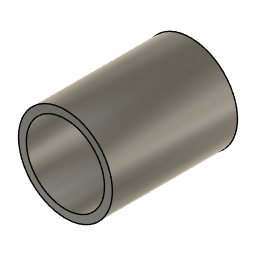
TANK v2 (Autodesk Fusion 360 archive; units mm, degrees)
design "Nozzle"
Autodesk Fusion 360 part; units mm, degrees
sketch "Sketch1" plane through (0, 0, 0) normal (0, 1, 0) x (1, 0, 0)
  circle A0 centre (0, 0) radius 12.5
  circle A1 centre (0, 0) radius 15
  dimension "d1" = 25
  dimension "d2" = 30
  constraint coincident A0.centre A1.centre
  constraint concentric A0 A1
  measures "d1" diameter of A0
  measures "d2" diameter of A1
extrude "Extrude1" add sketch "Sketch1" along normal blind 40

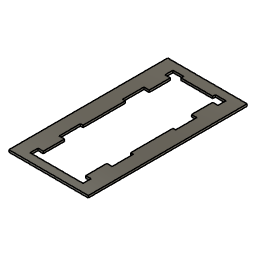
design "Potoboard holder"
Autodesk Fusion 360 part; units mm, degrees
sketch "Sketch1" plane through (0, 0, 0) normal (0, 0, 1) x (1, 0, 0)
  line L0 (-75, 150) -> (75, 150)
  line L1 (75, 150) -> (75, -150)
  line L2 (75, -150) -> (-75, -150)
  line L3 (-75, -150) -> (-75, 150)
  line L4 (-75, 150) -> (75, -150) construction
  line L5 (75, 150) -> (-75, -150) construction
  line L6 (50, 135) -> (-50, 135)
  line L7 (-50, 135) -> (-50, -135)
  line L8 (-50, -135) -> (50, -135)
  line L9 (50, -135) -> (50, 135)
  line L10 (50, 135) -> (-50, -135) construction
  line L11 (-50, 135) -> (50, -135) construction
  line L12 (-30, 135) -> (30, 135)
  line L13 (30, 135) -> (30, 130)
  line L14 (30, 130) -> (-30, 130)
  line L15 (-30, 130) -> (-30, 135)
  line L16 (-50, 40) -> (-45, 40)
  line L17 (-45, 40) -> (-45, -40)
  line L18 (-45, -40) -> (-50, -40)
  line L19 (-50, -40) -> (-50, 40)
  line L20 (-30, -135) -> (30, -135)
  line L21 (30, -135) -> (30, -130)
  line L22 (30, -130) -> (-30, -130)
  line L23 (-30, -130) -> (-30, -135)
  line L24 (50, 40) -> (45, 40)
  line L25 (45, 40) -> (45, -40)
  line L26 (45, -40) -> (50, -40)
  line L27 (50, -40) -> (50, 40)
  line L28 (-50, -80) -> (-40, -80)
  line L29 (-40, -80) -> (-40, -120)
  line L30 (-40, -120) -> (-50, -120)
  line L31 (-50, -120) -> (-50, -80)
  line L32 (50, -120) -> (40, -120)
  line L33 (40, -120) -> (40, -80)
  line L34 (40, -80) -> (50, -80)
  line L35 (50, -80) -> (50, -120)
  line L36 (50, 120) -> (40, 120)
  line L37 (40, 120) -> (40, 80)
  line L38 (40, 80) -> (50, 80)
  line L39 (50, 80) -> (50, 120)
  line L40 (-50, 120) -> (-40, 120)
  line L41 (-40, 120) -> (-40, 80)
  line L42 (-40, 80) -> (-50, 80)
  line L43 (-50, 80) -> (-50, 120)
  dimension "d1" = 300
  dimension "d2" = 150
  dimension "d3" = 270
  dimension "d4" = 100
  dimension "d5" = 60
  dimension "d6" = 20
  dimension "d7" = 5
  dimension "d8" = 80
  dimension "d9" = 95
  dimension "d10" = 5
  dimension "d11" = 60
  dimension "d12" = 5
  dimension "d13" = 20
  dimension "d14" = 80
  dimension "d15" = 5
  dimension "d16" = 95
  dimension "d19" = 10
  dimension "d20" = 40
  dimension "d21" = 40
  dimension "d22" = 10
  dimension "d23" = 40
  dimension "d24" = 40
  dimension "d25" = 10
  dimension "d26" = 40
  dimension "d27" = 40
  dimension "d28" = 10
  dimension "d29" = 40
  dimension "d30" = 40
  constraint horizontal L0
  constraint perpendicular L0 L1
  constraint parallel L0 L2
  constraint parallel L1 L3
  constraint coincident L4 origin
  constraint coincident L5 origin
  constraint horizontal L6
  constraint perpendicular L6 L7
  constraint parallel L6 L8
  constraint parallel L7 L9
  constraint coincident L10 origin
  constraint coincident L11 origin
  constraint horizontal L12
  constraint vertical L13
  constraint horizontal L14
  constraint vertical L15
  constraint coincident L6 L12.start
  constraint horizontal L16
  constraint vertical L17
  constraint horizontal L18
  constraint vertical L19
  constraint coincident L7 L16.start
  constraint horizontal L20
  constraint vertical L21
  constraint horizontal L22
  constraint vertical L23
  constraint coincident L8 L20.start
  constraint horizontal L24
  constraint vertical L25
  constraint horizontal L26
  constraint vertical L27
  constraint coincident L9 L24.start
  constraint horizontal L28
  constraint vertical L29
  constraint horizontal L30
  constraint vertical L31
  constraint coincident L7 L28.start
  constraint horizontal L32
  constraint vertical L33
  constraint horizontal L34
  constraint vertical L35
  constraint coincident L9 L32.start
  constraint horizontal L36
  constraint vertical L37
  constraint horizontal L38
  constraint vertical L39
  constraint coincident L9 L36.start
  constraint horizontal L40
  constraint vertical L41
  constraint horizontal L42
  constraint vertical L43
  constraint coincident L7 L40.start
  measures "d1" distance of L0.start L2.end
  measures "d2" distance of L0.start L0.end
  measures "d3" distance of L6.end L7.end
  measures "d4" distance of L6.start L6.end
  measures "d5" distance of L13.end L14.end
  measures "d6" distance of L6.end L12.start
  measures "d7" distance of L12.end L13.end
  measures "d8" distance of L16.end L17.end
  measures "d9" distance of L6.end L16.start
  measures "d10" distance of L17.end L18.end
  measures "d11" distance of L21.end L22.end
  measures "d12" distance of L20.start L22.end
  measures "d13" distance of L7.end L20.start
  measures "d14" distance of L24.end L25.end
  measures "d15" distance of L24.start L24.end
  measures "d16" distance of L6.start L24.start
  measures "d19" distance of L28.start L28.end
  measures "d20" distance of L28.end L29.end
  measures "d21" distance of L18.end L28.start
  measures "d22" distance of L32.start L32.end
  measures "d23" distance of L32.end L33.end
  measures "d24" distance of L26.end L34.end
  measures "d25" distance of L36.start L36.end
  measures "d26" distance of L36.end L37.end
  measures "d27" distance of L24 L38.end
  measures "d28" distance of L40.start L40.end
  measures "d29" distance of L40.end L41.end
  measures "d30" distance of L16.start L42.end
extrude "Extrude2" add sketch "Sketch1" along normal blind 4 contours L0 L1 L2 L3 | L6 L12 L13 L14 L15 | L9 L36 L37 L38 L39 | L9 L24 L25 L26 L27 | L7 L40 L41 L42 L43 | L9 L32 L33 L34 L35 | L7 L16 L17 L18 L19 | L7 L28 L29 L30 L31

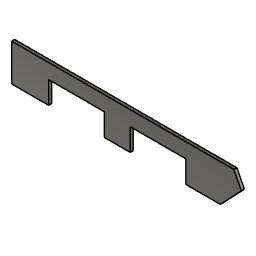
design "Side Plate"
Autodesk Fusion 360 part; units mm, degrees
sketch "Sketch1" plane through (0, 0, 0) normal (0, 1, 0) x (1, 0, 0)
  line L0 (0, 0) -> (0, -50)
  line L1 (0, -50) -> (300, -50)
  line L2 (0, 0) -> (50, 0)
  line L3 (50, 0) -> (50, -30)
  line L4 (50, -30) -> (125, -30)
  line L5 (125, -30) -> (125, 0)
  line L6 (125, 0) -> (160, 0)
  line L7 (160, 0) -> (160, -30)
  line L8 (160, -30) -> (235, -30)
  line L9 (235, -30) -> (235, 0)
  line L10 (235, 0) -> (281.5957, 0)
  line L11 (299.4269, -50.5394) -> (300, -50)
  line L12 (0, 0) -> (350, 0) construction
  line L13 (281.5957, 0) -> (310, -30) construction
  line L14 (310, -30) -> (300, -50) construction
  line L15 (281.5957, 0) -> (310, -30)
  line L16 (300, -50) -> (310, -30)
  dimension "d1" = 50
  dimension "d2" = 300
  dimension "d3" = 50
  dimension "d4" = 30
  dimension "d5" = 75
  dimension "d6" = 35
  dimension "d7" = 75
  dimension "d11" = 30
  dimension "d12" = 30
  dimension "d13" = 350
  dimension "d16" = 30
  dimension "d17" = 30
  dimension "d19" = 110
  dimension "d20" = 41.3135
  constraint coincident L0.start L2.start
  constraint vertical L0
  constraint perpendicular L0 L1
  constraint perpendicular L0 L2
  constraint perpendicular L2 L3
  constraint perpendicular L3 L4
  constraint perpendicular L4 L5
  constraint perpendicular L3 L6
  constraint perpendicular L6 L7
  constraint perpendicular L7 L8
  constraint perpendicular L8 L9
  constraint perpendicular L9 L10
  constraint perpendicular L0 L12
  measures "d1" distance of L0.start L0.end
  measures "d2" distance of L0.end L1.end
  measures "d3" distance of L0.start L2.end
  measures "d4" distance of L2.end L3.end
  measures "d5" distance of L3.end L4.end
  measures "d6" distance of L5.end L6.end
  measures "d7" distance of L7.end L8.end
  measures "d11" distance of L8.end L9.end
  measures "d12" distance of L6.end L7.end
  measures "d13" distance of L0.start L12.end
  measures "d16" distance of L4.end L5.end
  measures "d17" vertical distance of L10.end L13.end
  measures "d19" angle of L13 L14
  measures "d20" distance of L10.end L13.end
extrude "Extrude1" add sketch "Sketch1" along normal blind 4

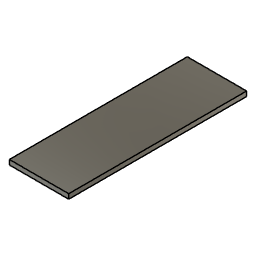
design "Back Board"
Autodesk Fusion 360 part; units mm, degrees
sketch "Sketch1" plane through (0, 0, 0) normal (0, 0, 1) x (1, 0, 0)
  line L0 (0, 0) -> (-50, 0)
  line L1 (-50, 0) -> (-50, 150)
  line L2 (-50, 150) -> (0, 150)
  line L3 (0, 150) -> (0, 0)
  dimension "d1" = 150
  dimension "d2" = 50
  constraint horizontal L0
  constraint vertical L1
  constraint horizontal L2
  constraint vertical L3
  constraint coincident L0.start L3.end
  measures "d1" distance of L0.start L2.end
  measures "d2" distance of L0.start L0.end
extrude "Extrude1" add sketch "Sketch1" along normal blind 4

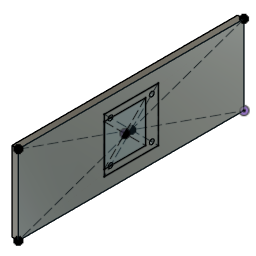
design "Untitled"
Autodesk Fusion 360 part; units mm, degrees
sketch "Sketch1" plane through (0, 0, 0) normal (1, 0, 0) x (0, 1, 0)
  line L0 (0, 0) -> (-142, 0)
  line L1 (-142, 0) -> (-142, 50)
  line L2 (-142, 50) -> (0, 50)
  line L3 (0, 50) -> (0, 0)
  dimension "d1" = 142
  dimension "d2" = 50
  constraint horizontal L0
  constraint vertical L1
  constraint horizontal L2
  constraint vertical L3
  constraint coincident L0.start L3.end
  measures "d1" distance of L1.end L2.end
  measures "d2" distance of L0.start L2.end
extrude "Extrude1" add sketch "Sketch1" along normal blind 4
sketch "Sketch2" plane through (4, 0, 0) normal (1, 0, 0) x (0, 1, 0)
  line L0 (0, 50) -> (-142, 50)
  line L1 (-142, 50) -> (-142, 0)
  line L2 (-142, 0) -> (0, 0)
  line L3 (0, 0) -> (0, 50)
  line L4 (-142, 50) -> (0, 0) construction
  line L5 (0, 50) -> (-142, 0) construction
  line L6 (-54, 42) -> (-88, 42) construction
  line L7 (-88, 42) -> (-88, 8) construction
  line L8 (-88, 8) -> (-54, 8) construction
  line L9 (-54, 8) -> (-54, 42) construction
  line L10 (-54, 42) -> (-88, 8) construction
  line L11 (-88, 42) -> (-54, 8) construction
  line L12 (-88, 42) -> (-54, 42)
  line L13 (-54, 42) -> (-54, 8)
  line L14 (-54, 8) -> (-88, 8)
  line L15 (-88, 8) -> (-88, 42)
  point P0 (-71, 25)
  dimension "d5" = 34
  dimension "d6" = 34
  constraint coincident L0.end L1.start
  constraint coincident L2.end L3.start
  constraint coincident L0.start L3.end
  constraint coincident L1.end L2.start
  constraint horizontal L6
  constraint perpendicular L6 L7
  constraint parallel L6 L8
  constraint parallel L7 L9
  constraint coincident L10 P0
  constraint coincident L11 P0
  constraint midpoint L4 P0
  constraint horizontal L12
  constraint vertical L13
  constraint horizontal L14
  constraint vertical L15
  measures "d5" distance of L7.end L8.end
  measures "d6" distance of L6.end L7.end
sketch "Sketch3" plane through (4, -75, 25) normal (1, 0, 0) x (0, 1, 0)
  line L0 (13, 13) -> (-13, 13)
  line L1 (-13, 13) -> (-13, -13)
  line L2 (-13, -13) -> (13, -13)
  line L3 (13, -13) -> (13, 13)
  line L4 (13, 13) -> (-13, -13) construction
  line L5 (-13, 13) -> (13, -13) construction
  dimension "d7" = 26
  dimension "d8" = 26
  constraint horizontal L0
  constraint perpendicular L0 L1
  constraint parallel L0 L2
  constraint parallel L1 L3
  constraint coincident L4 origin
  constraint coincident L5 origin
  measures "d7" distance of L1.end L2.end
  measures "d8" distance of L0.end L1.end
sketch "Sketch4" plane through (4, 0, 0) normal (1, 0, 0) x (0, 1, 0)
  circle A0 centre (-84, 38) radius 1.5
  circle A1 centre (-58, 38) radius 1.5
  circle A2 centre (-84, 12) radius 1.5
  circle A3 centre (-58, 12) radius 1.5
  line L0 (-88, 42) -> (-54, 42)
  line L1 (-54, 8) -> (-88, 8)
  line L2 (-88, 8) -> (-88, 42)
  line L3 (-54, 42) -> (-54, 8)
  line L4 (-54, 42) -> (-88, 42)
  dimension "d9" = 3
  dimension "d10" = 3
  dimension "d11" = 3
  dimension "d12" = 3
  dimension "d13" = 26
  dimension "d14" = 26
  dimension "d15" = 26
  dimension "d16" = 26
  dimension "d17" = 4
  dimension "d18" = 4
  dimension "d19" = 4
  dimension "d20" = 4
  dimension "d21" = 4
  dimension "d22" = 4
  measures "d9" diameter of A0
  measures "d10" diameter of A1
  measures "d11" diameter of A2
  measures "d12" diameter of A3
  measures "d13" distance of A1.centre A3.centre
  measures "d14" distance of A2.centre A3.centre
  measures "d15" distance of A0.centre A2.centre
  measures "d16" distance of A0.centre A1.centre
  measures "d17" distance of A0.centre L0
  measures "d18" distance of A2.centre L1
  measures "d19" distance of A0.centre L2
  measures "d20" distance of A2.centre L2
  measures "d21" distance of A3.centre L3
  measures "d22" distance of A1.centre L4
extrude "Extrude2" cut sketch "Sketch4" against normal through all contours A0 | A1 | A2 | A3
